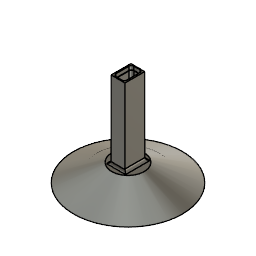
SensorHolder (Autodesk Fusion 360 design; units mm, degrees)
Autodesk Fusion 360 part; units mm, degrees
sketch "Sketch1" plane through (0, 0, 0) normal (0, 0, 1) x (1, 0, 0)
  line L0 (1.25, -4.4) -> (3.95, -4.4)
  line L1 (5.2, -3.15) -> (5.2, 3.05)
  line L2 (3.95, 4.3) -> (1.25, 4.3)
  line L3 (0, 3.05) -> (0, -3.15)
  arc A0 (1.25, 4.3) -> (0, 3.05) centre (1.25, 3.05) ccw
  arc A1 (0, -3.15) -> (1.25, -4.4) centre (1.25, -3.15) ccw
  arc A2 (5.2, 3.05) -> (3.95, 4.3) centre (3.95, 3.05) ccw
  arc A3 (3.95, -4.4) -> (5.2, -3.15) centre (3.95, -3.15) ccw
  point P0 (0, 4.3)
  dimension "d2" = 4.3
  dimension "d4" = 1.25
  dimension "d32" = 5.2
  dimension "d38" = 8.7
  constraint horizontal L0
  constraint vertical L1
  constraint horizontal L2
  constraint vertical L3
  constraint coincident P0 L2
  constraint coincident P0 L3
  constraint tangent L2 A0
  constraint tangent L3 A0
  measures "d2" distance of origin P0
  measures "d4" radius of A0
  measures "d32" distance of L1 L3
  measures "d38" distance of L0 L2
extrude "Extrude1" add sketch "Sketch1" along normal blind 48 makes body 1
sketch "Sketch2" plane through (0, 0, 48) normal (0, 0, 1) x (-1, 0, 0)
  arc A0 (-3.95, 4.4) -> (-5.2, 3.15) centre (-3.95, 3.15) ccw
  line L0 (-5.2, 3.15) -> (-5.2, -3.05)
  arc A1 (-5.2, -3.05) -> (-3.95, -4.3) centre (-3.95, -3.05) ccw
  line L1 (-3.95, -4.3) -> (-1.25, -4.3)
  arc A2 (-1.25, -4.3) -> (0, -3.05) centre (-1.25, -3.05) ccw
  line L2 (0, -3.05) -> (0, 3.15)
  arc A3 (0, 3.15) -> (-1.25, 4.4) centre (-1.25, 3.15) ccw
  line L3 (-1.25, 4.4) -> (-3.95, 4.4)
  line L4 (-1.0576, 4.6824) -> (-4.147, 4.6768)
  line L5 (-5.4, 3.4215) -> (-5.4, -3.2435)
  line L6 (-4.1383, -4.4987) -> (-1.0488, -4.4829)
  line L7 (0.2, -3.2276) -> (0.2, 3.4272)
  arc A4 (-1.0488, -4.4829) -> (0.2, -3.2276) centre (-1.0553, -3.2276) ccw
  arc A5 (-5.4, -3.2435) -> (-4.1383, -4.4987) centre (-4.1447, -3.2435) ccw
  arc A6 (-4.147, 4.6768) -> (-5.4, 3.4215) centre (-4.1447, 3.4215) ccw
  arc A7 (0.2, 3.4272) -> (-1.0576, 4.6824) centre (-1.0553, 3.4272) ccw
  line L8 (-2.5094, -4.8914) -> (0.8801, -4.8914)
  line L9 (0.8801, -4.8914) -> (0.8801, 5.1292)
  line L10 (0.8801, 5.1292) -> (-6.1692, 5.1292)
  line L11 (-6.1692, 5.1292) -> (-6.1709, -4.8908)
  line L12 (-6.1709, -4.8908) -> (-2.5094, -4.8914)
  point P0 (-2.5, -2.15)
  dimension "d35" = 0.2
  dimension "d36" = 0.2
  constraint parallel L5 L7
  constraint tangent L6 A4
  constraint tangent L7 A4
  constraint tangent L5 A5
  constraint tangent L6 A5
  constraint equal A4 A5
  constraint tangent L4 A6
  constraint tangent L5 A6
  constraint equal A4 A6
  constraint tangent L4 A7
  constraint tangent L7 A7
  constraint equal A4 A7
  constraint perpendicular L11 L12
  measures "d35" distance of L0 L5
  measures "d36" distance of L2 L7
extrude "Extrude2" add sketch "Sketch2" against normal blind 48 separate body contours L8 L9 L10 L11 L12 makes body 2
sketch "Sketch4" plane through (0, 0, 0) normal (0, 0, -1) x (1, 0, 0)
  arc A0 (5.2, 3.15) -> (3.95, 4.4) centre (3.95, 3.15) ccw
  line L0 (3.95, 4.4) -> (1.25, 4.4)
  arc A1 (1.25, 4.4) -> (0, 3.15) centre (1.25, 3.15) ccw
  line L1 (0, 3.15) -> (0, -3.05)
  arc A2 (0, -3.05) -> (1.25, -4.3) centre (1.25, -3.05) ccw
  line L2 (1.25, -4.3) -> (3.95, -4.3)
  arc A3 (3.95, -4.3) -> (5.2, -3.05) centre (3.95, -3.05) ccw
  line L3 (5.2, -3.05) -> (5.2, 3.15)
  line L4 (5.4558, -4.5722) -> (-0.271, -4.5722)
  line L5 (-0.271, -4.5722) -> (-0.271, 4.8144)
  line L6 (-0.271, 4.8144) -> (5.4558, 4.8144)
  line L7 (5.4558, 4.8144) -> (5.4558, -4.5722)
  constraint horizontal L4
  constraint vertical L5
  constraint horizontal L6
  constraint vertical L7
extrude "Extrude3" add sketch "Sketch4" against normal blind 46.1 separate body makes body 3
combine "Combine1" operation add target body 2 tool bodies 3
sketch "Sketch5" plane through (0, 0, 0) normal (0, 1, 0) x (1, 0, 0)
  line L0 (-0.4775, 0) -> (-0.2775, 0)
  line L1 (5.5663, 0) -> (5.4646, 0)
  line L2 (5.4646, 0) -> (-0.2775, 0)
  line L3 (-0.2775, 0) -> (-0.2775, -23)
  line L4 (-0.2775, -23) -> (5.4646, -23)
  line L5 (5.4646, -23) -> (5.4646, 0)
  line L6 (5.6646, 0) -> (5.4646, 0)
  dimension "d16" = 0.2
  dimension "d39" = 0.2
  constraint horizontal L0
  constraint horizontal L1
  constraint perpendicular L2 L3
  constraint parallel L2 L4
  constraint parallel L3 L5
  constraint parallel L0 L2
  constraint parallel L1 L6
  measures "d16" distance of L0.start L0.end
  measures "d39" distance of L6.start L1.end
extrude "Extrude4" cut sketch "Sketch5" along normal blind 6 and the other way blind 2 bodies 2
sketch "Sketch6" plane through (0, 0, 0) normal (0, 0, 1) x (1, 0, 0)
  line L0 (-0.3357, 4.8248) -> (5.6703, 4.8248)
  line L1 (5.6703, 4.8248) -> (2.6673, 4.8248)
  line L2 (2.6673, 4.8248) -> (2.6673, -5.0358)
  circle A0 centre (2.6673, -0.1055) radius 25
  circle A1 centre (2.6673, -0.1055) radius 27.5
  dimension "d22" = 50
  dimension "d29" = 55
  constraint horizontal L0
  constraint midpoint L0 L1.end
  constraint perpendicular L1 L2
  constraint midpoint L2 A0.centre
  constraint concentric A0 A1
  measures "d22" diameter of A0
  measures "d29" diameter of A1
extrude "Extrude5" add sketch "Sketch6" along normal blind 9 draft -65 contours A0 | A1 bodies 2
fillet "Fillet1" radius 1.3 tangency weight 0.78388 4 edges at (-0.8801, -0.1189, 9) (5.8177, 4.8909, 9) (-0.5788, 4.8914, 9) (6.17, -0.1192, 9) on bodies 2
fillet "Fillet2" radius 1 tangency weight 0.71642 8 edges at (0.3661, -4.0339, 9) (0, -2.575, 9) (2.6, -4.4, 9) (4.8339, -4.0339, 9) (5.2, -2.575, 9) (-0.2775, 2.0957, 9) (5.4646, 2.0955, 9) (2.6445, -5.1292, 9) on bodies 2
extrude "Extrude6" cut sketch "Sketch6" along normal blind 5 draft -62 contours A0 bodies 2
hidden bodies 1
